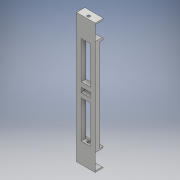
# Autodesk Inventor part: Raket_Lednings_Holder_Mindre
Saved by Autodesk Inventor 2018 (Build 220112000, 112)
## iProperties
Created: 2017-08-14
Part Number: Raket_Lednings_Holder_Mindre
Material: Generic
Document SubType Name: Modeling
Designer: andre
Density: 1 g/cm^3
Appearance: Default
Author: andre
## iProperties of the stored document Raket_Lednings_Holder_3DPrint.ipt
Created: 2017-08-14
Part Number: Raket_Lednings_Holder_3DPrint
Material: Generic
Document SubType Name: Modeling
Designer: andre
Density: 1 g/cm^3
Appearance: Default
Author: andre
Autodesk Inventor part; units mm, degrees
ref_plane "YZ Plane" through (0, 0, 0) normal (1, 0, 0) x (0, 1, 0)
ref_plane "XZ Plane" through (0, 0, 0) normal (0, 1, 0) x (-1, 0, 0)
ref_plane "XY Plane" through (0, 0, 0) normal (0, 0, 1) x (1, 0, 0)
sketch "Sketch1" plane through (0, 0, 0) normal (0, 1, 0) x (-1, 0, 0)
  line L0 (0, 0) -> (20, 0)
  line L1 (20, 0) -> (20, -140)
  line L2 (20, -140) -> (0, -140)
  line L3 (0, -140) -> (0, 0)
  dimension "d0" = 20
  dimension "d1" = 140
  constraints: 8 end point, 2 parallel, 1 horizontal, 1 perpendicular
  measures "d0" distance of L1.end L2.end
  measures "d1" distance of L0.end L1.end
extrude "Extrusion1" add sketch "Sketch1" along normal blind 5
sketch "Sketch2" plane through (0, 5, 0) normal (0, 1, 0) x (1, 0, 0)
  line L0 (0, 0) -> (0, 140) projected
  line L1 (-20, 140) -> (-20, 0) projected
  line L2 (0, 0) -> (-20, 0)
  line L3 (-20, 0) -> (-20, 20)
  line L4 (-20, 20) -> (0, 20)
  line L5 (0, 20) -> (0, 0)
  line L6 (-20, 140) -> (0, 140)
  line L7 (0, 140) -> (0, 120)
  line L8 (0, 120) -> (-20, 120)
  line L9 (-20, 120) -> (-20, 140)
  dimension "d4" = 20
  dimension "d5" = 20
  constraints: 16 end point, 4 parallel, 2 horizontal, 2 perpendicular, 2 point on line
  measures "d4" distance of L2.end L3.end
  measures "d5" distance of L6.end L7.end
extrude "Extrusion2" add sketch "Sketch2" along normal blind 4 contours L2 L1 L4 L0 | L8 L1 L6 L0
sketch "Sketch3" plane through (0, 9, 0) normal (0, 1, 0) x (1, 0, 0)
  line L0 (0, 0) -> (0, 5)
  line L1 (0, 0) -> (0, 20) projected
  line L2 (0, 5) -> (0, 15)
  line L3 (-20, 20) -> (-20, 0) projected
  line L4 (0, 13.8957) -> (-20, 13.8957)
  line L5 (-20, 13.8957) -> (-20, 5)
  line L6 (-20, 5) -> (0, 5)
  line L7 (0, 5) -> (0, 13.8957)
  line L8 (0, 140) -> (0, 0) projected
  line L9 (0, 140) -> (0, 135)
  line L10 (0, 135) -> (0, 125)
  line L11 (-20, 0) -> (-20, 140) projected
  line L12 (0, 125) -> (-20, 125)
  line L13 (-20, 140) -> (0, 140)
  line L14 (-20, 125) -> (-20, 140)
  line L15 (0, 135) -> (-20, 135)
  point P0 (-20, 195)
  dimension "d8" = 5
  dimension "d9" = 10
  dimension "d10" = 5
  dimension "d11" = 10
  constraints: 24 end point, 8 point on line, 4 horizontal, 2 parallel, 1 collinear, 1 perpendicular
  measures "d8" distance of L0.start L0.end
  measures "d9" distance of L0.end L2.end
  measures "d10" distance of L8.start L9.end
  measures "d11" distance of L9.end L10.end
extrude "Extrusion3" cut sketch "Sketch3" against normal blind 5 contours L6 L3 L4 L1 | L12 L11 L15 L8
sketch "Sketch4" plane through (0, 0, 0) normal (1, 0, 0) x (0, 0, -1)
  line L0 (13.8957, 4) -> (5, 4) projected
  line L1 (5, 4) -> (5, 0)
  line L2 (0, 0) -> (140, 0) projected
  line L3 (5, 2) -> (200, 2)
  circle A0 centre (9.4478, 2) radius 1
  circle A1 centre (130, 2) radius 1
  dimension "d46" = 2
  dimension "d60" = 2
  constraints: 4 end point, 3 point on line, 2 centre point, 1 midpoint, 1 perpendicular, 1 vertical
  measures "d46" diameter of A0
  measures "d60" diameter of A1
extrude "Extrusion4" cut sketch "Sketch4" against normal blind 50
sketch "Sketch5" plane through (0, 5, 0) normal (0, 1, 0) x (1, 0, 0)
  line L0 (0, 20) -> (-20, 20) projected
  line L1 (-20, 20) -> (-20, 22)
  line L2 (-20, 0) -> (-20, 140) projected
  line L3 (-20, 22) -> (-15, 22)
  line L4 (0, 120) -> (0, 118)
  line L5 (0, 118) -> (-5, 118)
  line L6 (-15, 22) -> (-5, 22)
  line L7 (-5, 22) -> (-5, 118)
  line L8 (-5, 118) -> (-15, 118)
  line L9 (-15, 118) -> (-15, 22)
  line L10 (-15, 70) -> (-15, 72.5)
  line L11 (-15, 72.5) -> (-5, 72.5)
  line L12 (-5, 72.5) -> (-5, 67.5)
  line L13 (-5, 67.5) -> (-15, 67.5)
  line L14 (-15, 67.5) -> (-15, 72.5)
  line L15 (-5, 67.5) -> (-5, 62.5)
  line L16 (-5, 72.5) -> (-5, 77.5)
  line L17 (-5, 62.5) -> (-15, 62.5)
  line L18 (-15, 62.5) -> (-15, 22)
  line L19 (-15, 22) -> (-5, 22)
  line L20 (-5, 22) -> (-5, 62.5)
  line L21 (-5, 77.5) -> (-15, 77.5)
  line L22 (-15, 77.5) -> (-15, 118)
  line L23 (-15, 118) -> (-5, 118)
  line L24 (-5, 118) -> (-5, 77.5)
  point P0 (0, 0)
  dimension "d17" = 2
  dimension "d18" = 5
  dimension "d19" = 2
  dimension "d21" = 5
  dimension "d22" = 2.5
  dimension "d23" = 5
  dimension "d24" = 5
  dimension "d25" = 5
  constraints: 46 end point, 8 parallel, 5 horizontal, 5 perpendicular, 5 point on line, 1 midpoint
  measures "d17" distance of L0.end L1.end
  measures "d18" distance of L1.end L3.end
  measures "d19" distance of L4.start L4.end
  measures "d21" distance of L4.end L5.end
  measures "d22" distance of L10.start L10.end
  measures "d23" distance of L11.end L12.end
  measures "d24" distance of L12.end L15.end
  measures "d25" distance of L11.end L16.end
extrude "Extrusion5" cut sketch "Sketch5" against normal blind 10 contours L9 L17 L7 L6 | L9 L11 L7 L13 | L21 L9 L8 L7
chamfer "Chamfer1" distance 4 angle 45 4 edges at (0, 4, -9.4478) (0, 4, -130) (-20, 4, -130) (-20, 4, -9.4478)
chamfer "Chamfer2" distance 5 angle 45 4 edges at (-10, 9, -13.8957) (-10, 9, -125) (-10, 9, -5) (-10, 9, -135)
chamfer "Chamfer3" distance 3.5 angle 45 8 edges at (0, 2.0001, -125) (0, 2, -5) (-20, 2, -5) (-20, 2.0001, -125) (-20, 2, -13.8957) (0, 2, -13.8957) (-20, 2, -135) (0, 2, -135)
sketch "Sketch8" plane through (0, 0, -140) normal (0, 0, -1) x (-1, 0, 0)
  line L0 (20, 0) -> (0, 0) projected
  line L1 (10, 0) -> (10, 3)
  circle A0 centre (10, 3) radius 1.5
  dimension "d53" = 3
  dimension "d54" = 3
  constraints: 2 end point, 1 centre point, 1 coincident, 1 midpoint, 1 vertical
  measures "d53" distance of L1.start L1.end
  measures "d54" diameter of A0
extrude "Extrusion8" cut sketch "Sketch8" against normal blind 30
sketch "Sketch9" plane through (-20, 0, 0) normal (0, 0, 1) x (1, 0, 0)
  line L0 (15, 0) -> (5, 0) projected
  line L1 (10, 0) -> (10, 5)
  circle A0 centre (10, 3) radius 1.5 projected
  circle A1 centre (10, 3) radius 1.5
  point P0 (20, 0)
  dimension "d57" = 5
  constraints: 2 end point, 1 centre point, 1 coincident, 1 midpoint, 1 vertical
  measures "d57" distance of L1.start L1.end
extrude "Extrusion9" cut sketch "Sketch9" against normal blind 30
chamfer "Chamfer4" distance 3 angle 45 1 edges at (-4, 4, -130)
chamfer "Chamfer5" distance 3 angle 45 3 edges at (-16, 4, -130) (-4, 4, -9.4478) (-16, 4, -9.4478)
body "Solid1"
